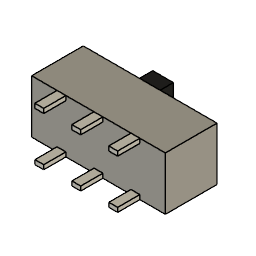
olliebella v1 extended (Autodesk Fusion 360 archive; units mm, degrees)
design "MSK-1153 slide switch SLV"
Autodesk Fusion 360 part; units mm, degrees
note: some values were not read from the file. Chosen so that the rebuilt part matches the saved one: which bodies a step acts on; which face or edge a step refers to.
sketch "Sketch1" plane through (0, 0, 0) normal (0, 0, 1) x (1, 0, 0)
  line L0 (-4.525, 3.5) -> (4.525, 3.5)
  line L1 (4.525, 3.5) -> (4.525, 0)
  line L2 (4.525, 0) -> (-4.525, 0)
  line L3 (-4.525, 0) -> (-4.525, 3.5)
  line L4 (-1.825, 5.5) -> (-0.425, 5.5)
  line L5 (-0.425, 5.5) -> (-0.425, 3.5)
  line L6 (-0.425, 3.5) -> (-1.825, 3.5)
  line L7 (-1.825, 3.5) -> (-1.825, 5.5)
  line L8 (-4.525, 0) -> (-4.525, -3.1) construction
  line L9 (-4.525, -3.1) -> (4.525, -3.1) construction
  line L10 (4.525, -3.1) -> (4.525, 0) construction
  line L11 (0, 0) -> (0, -3.1) construction
  line L12 (0.3, 0) -> (0.3, -3.1)
  line L13 (-0.3, -3.1) -> (-0.3, 0)
  line L14 (0.3, -1.55) -> (-0.3, -1.55) construction
  line L15 (-0.3, -3.1) -> (0.3, -3.1)
  line L16 (-2.8, 0) -> (-2.8, -3.1)
  line L17 (-2.2, -3.1) -> (-2.2, 0)
  line L18 (-2.5, 0) -> (-2.5, -3.1) construction
  line L19 (-2.8, -3.1) -> (-2.2, -3.1)
  line L20 (-2.8, -1.55) -> (-2.2, -1.55) construction
  line L21 (2.5, 0) -> (2.5, -3.1) construction
  line L22 (2.8, 0) -> (2.8, -3.1)
  line L23 (2.2, -3.1) -> (2.2, 0)
  line L24 (2.2, -1.55) -> (2.8, -1.55) construction
  line L25 (2.8, -3.1) -> (2.2, -3.1)
  line L26 (-2.025, 3.5) -> (-2.025, 2.9)
  line L27 (-2.025, 2.9) -> (2.025, 2.9)
  line L28 (2.025, 2.9) -> (2.025, 3.5)
  line L29 (-0.425, 5.5) -> (1.825, 5.5) construction
  line L30 (1.825, 5.5) -> (1.825, 3.5) construction
  dimension "d1" = 9.05
  dimension "d2" = 3.5
  dimension "d3" = 2
  dimension "d4" = 1.4
  dimension "d5" = 2.7
  dimension "d6" = 6.6
  dimension "d7" = 0.6
  dimension "d8" = 2.5
  dimension "d9" = 2.5
  dimension "d24" = 0.6
  dimension "d25" = 0.2
  dimension "d26" = 2.7
  dimension "d27" = 0.2
  constraint horizontal L0
  constraint vertical L1
  constraint horizontal L2
  constraint vertical L3
  constraint midpoint L11.start L2
  constraint horizontal L4
  constraint vertical L5
  constraint horizontal L6
  constraint vertical L7
  constraint coincident L0 L5.end
  constraint perpendicular L2 L8
  constraint perpendicular L1 L9
  constraint perpendicular L2 L10
  constraint coincident L11.start origin
  constraint midpoint L9 L11.end
  constraint coincident L2 L12.start
  constraint coincident L9 L12.end
  constraint coincident L9 L13.start
  constraint coincident L2 L13.end
  constraint vertical L13
  constraint vertical L12
  constraint midpoint L12 L14.start
  constraint midpoint L13 L14.end
  constraint midpoint L11 L14
  constraint coincident L2 L16.start
  constraint coincident L9 L16.end
  constraint coincident L9 L17.start
  constraint coincident L2 L17.end
  constraint vertical L17
  constraint vertical L16
  constraint coincident L2 L18.start
  constraint coincident L9 L18.end
  constraint perpendicular L9 L18
  constraint midpoint L16 L20.start
  constraint midpoint L17 L20.end
  constraint equal L14 L20
  constraint midpoint L18 L20
  constraint coincident L2 L21.start
  constraint coincident L9 L21.end
  constraint perpendicular L9 L21
  constraint coincident L2 L22.start
  constraint coincident L9 L22.end
  constraint coincident L9 L23.start
  constraint coincident L2 L23.end
  constraint vertical L23
  constraint vertical L22
  constraint midpoint L23 L24.start
  constraint midpoint L22 L24.end
  constraint midpoint L21 L24
  constraint equal L14 L24
  constraint coincident L0 L26.start
  constraint perpendicular L0 L26
  constraint perpendicular L26 L27
  constraint coincident L0 L28.end
  constraint perpendicular L0 L28
  constraint perpendicular L5 L29
  constraint coincident L0 L30.end
  constraint perpendicular L0 L30
  measures "d1" distance of L0.start L0.end
  measures "d2" distance of L0.start L2.end
  measures "d3" distance of L4 L6
  measures "d4" distance of L5 L7
  measures "d5" distance of L0.start L7
  measures "d6" distance of L0 L9
  measures "d7" distance of L14.start L14.end
  measures "d8" distance of L11 L18
  measures "d9" distance of L11 L21
  measures "d24" distance of L0 L27
  measures "d25" distance of L7 L26
  measures "d26" distance of L0.end L30
  measures "d27" distance of L28 L30
extrude "Extrude2" add sketch "Sketch1" along normal blind 1.8 and the other way blind 1.8 contours L0 L1 L2 L3 L26 L27 L28 | L0 L6 L26 L27 L28 makes body 1
extrude "Extrude1" add sketch "Sketch1" against normal blind 0.3 from surface at 1.8 separate body contours L2 L16 L17 L19 | L2 L12 L13 L15 | L2 L22 L23 L25 makes body 2 at (-2.6, -1.0333, 1.8) makes body 3 at (-0.1, -1.0333, 1.8) makes body 4 at (2.4, -1.0333, 1.8)
extrude "Extrude3" add sketch "Sketch1" along normal blind 0.3 from surface at -1.8 separate body contours L2 L16 L17 L19 | L2 L12 L13 L15 | L2 L22 L23 L25 makes body 5 at (-2.6, -1.0333, -1.8) makes body 6 at (-0.1, -1.0333, -1.8) makes body 7 at (2.4, -1.0333, -1.8)
extrude "Extrude4" add sketch "Sketch1" along normal blind 0.7 and the other way blind 0.7 separate body contours L0 L4 L5 L6 L7 makes body 8
extrude "Extrude5" add sketch "Sketch1" along normal up to surface (0.9 mm away) and the other way up to surface (0.9 mm away) separate body contours L0 L6 L26 L27 L28 makes body 9
combine "Combine1" operation cut target body 1 tool bodies 9 keep tools
move_body "Move1" bodies 9 to x (1, 0, 0) y (0, 1, 0) z (0, 0, 1) at (0, -0.2, 0)
extrude "Extrude6" add 1 faces at (-1.3583, 3.5, -0.2333) along direction (0, -1, 0) blind 0.5 on bodies 8 bodies 8 9
extrude "Extrude7" cut 1 faces at (-1.5083, 0, 0.6) along direction (0, -1, 0) up to surface (1.6 mm away) from surface at 1.5 on bodies 1 bodies 2 3 4 5 6 7

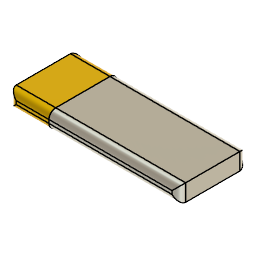
design "Lipo 100mAh 301230"
Autodesk Fusion 360 part; units mm, degrees
sketch "Sketch1" plane through (0, 0, 0) normal (0, 0, 1) x (1, 0, 0) in component "Lipo_Body"
  line L0 (15, -6) -> (-15, -6)
  line L1 (-15, -6) -> (-15, 6)
  line L2 (-15, 6) -> (15, 6)
  line L3 (15, 6) -> (15, -6)
  line L4 (15, -6) -> (-15, 6) construction
  line L5 (-15, -6) -> (15, 6) construction
  line L6 (-8, 6) -> (-8, -6)
  dimension "d1" = 30
  dimension "d3" = 7
  dimension "d74" = 12
  constraint horizontal L0
  constraint perpendicular L0 L1
  constraint parallel L0 L2
  constraint parallel L1 L3
  constraint coincident L4 origin
  constraint coincident L5 origin
  constraint coincident L2 L6.start
  constraint coincident L0 L6.end
  constraint perpendicular L0 L6
  measures "d1" distance of L1.end L2.end
  measures "d3" distance of L1 L6
  measures "d74" distance of L0 L2
extrude "Extrude1" add sketch "Sketch1" along normal blind 3 contours L0 L2 L3 L6 makes body 1 in component "Lipo_Body"
extrude "Extrude2" add sketch "Sketch1" along normal up to surface (3 mm away) separate body contours L0 L1 L2 L6 makes body 2 in component "Lipo_Body"
fillet "Fillet1" radius 1.2 12 edges at (15, -6, 1.5) (15, 6, 1.5) (3.5, -6, 3) (3.5, -6, 0) (3.5, 6, 3) (3.5, 6, 0) (-15, -6, 1.5) (-15, 6, 1.5) (-11.5, -6, 3) (-11.5, -6, 0) (-11.5, 6, 3) (-11.5, 6, 0) on bodies 1 2 in component "Lipo_Body"
shell "Shell2" [suppressed] in component "Lipo_Body"
component "Lipo_Body" placed x (1, 0, 0) y (0, 1, 0) z (0, 0, 1) at (0, 0, 0)
equation "d5_1 = 0.1 mm + 0.05 mm"
equation "d9_1 = 0.1 mm - 0.05 mm"
equation "d13_1 = ( 2.8 / 2 ) * 1 mm"
equation "d19_1 = ( 1.9 / 2 ) * 1 mm"
equation "d20_1 = ( -1.9 / 2 ) * 1 mm"
equation "d13_2 = ( 2.8 / 2 ) * 1 mm"
equation "d19_2 = ( 1.9 / 2 ) * 1 mm"
equation "d20_2 = ( -1.9 / 2 ) * 1 mm"
equation "d80 = 1.6 mm - 0.3 mm"
named bodies: "sticker"

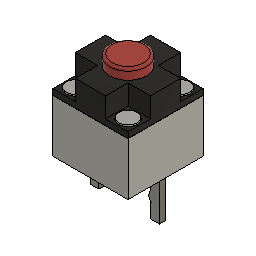
design "kailh cmi627301D07"
Autodesk Fusion 360 part; units mm, degrees
ref_plane "WorkPlane1" through (0, 0, 10) normal (0, 0, 1) x (1, 0, 0)
ref_plane "WorkPlane2" through (0, 0, 3.5) normal (0, 0, 1) x (1, 0, 0)
ref_plane "WorkPlane3" through (0, 0, 0.2) normal (0, 0, 1) x (1, 0, 0)
sketch "top" plane through (0, 0, 10) normal (0, 0, 1) x (1, 0, 0)
  line L0 (0, 0) -> (0, 5) construction
  line L1 (3.1, 8.1) -> (-3.1, 8.1)
  line L2 (-3.1, 8.1) -> (-3.1, 1.9)
  line L3 (-3.1, 1.9) -> (3.1, 1.9)
  line L4 (3.1, 1.9) -> (3.1, 8.1)
  line L5 (3.1, 8.1) -> (-3.1, 1.9) construction
  line L6 (-3.1, 8.1) -> (3.1, 1.9) construction
  circle A0 centre (0, 5) radius 1.5
  line L7 (-3.1, 6.25) -> (3.1, 6.25) construction
  line L8 (3.1, 3.75) -> (-3.1, 3.75) construction
  line L9 (-1.25, 8.1) -> (-1.25, 1.9) construction
  line L10 (1.25, 1.9) -> (1.25, 8.1) construction
  line L11 (1.25, 6.25) -> (-1.25, 3.75) construction
  line L12 (-1.25, 8.1) -> (-1.25, 6.25)
  line L13 (-3.1, 6.25) -> (-1.25, 6.25)
  line L14 (1.25, 6.25) -> (1.25, 8.1)
  line L15 (1.25, 6.25) -> (3.1, 6.25)
  line L16 (1.25, 3.75) -> (3.1, 3.75)
  line L17 (1.25, 3.75) -> (1.25, 1.9)
  line L18 (-1.25, 3.75) -> (-1.25, 1.9)
  line L19 (-1.25, 3.75) -> (-3.1, 3.75)
  line L20 (1.25, 3.75) -> (3.1, 1.9) construction
  line L21 (1.25, 6.25) -> (3.1, 8.1) construction
  line L22 (-1.25, 6.25) -> (-3.1, 8.1) construction
  line L23 (-1.25, 3.75) -> (-3.1, 1.9) construction
  circle A1 centre (2.175, 2.825) radius 0.75
  circle A2 centre (-2.175, 2.825) radius 0.75
  circle A3 centre (-2.175, 7.175) radius 0.75
  circle A4 centre (2.175, 7.175) radius 0.75
  point P0 (0, 5)
  dimension "d3" = 5
  dimension "d4" = 6.2
  dimension "d5" = 6.2
  dimension "d6" = 3
  dimension "d7" = 2.5
  dimension "d8" = 2.5
  dimension "d19" = 1.5
  constraint coincident L0.start origin
  constraint vertical L0
  constraint horizontal L1
  constraint perpendicular L1 L2
  constraint parallel L1 L3
  constraint parallel L2 L4
  constraint coincident L5 P0
  constraint coincident L6 P0
  constraint coincident P0 L0.end
  constraint coincident L2 L7.start
  constraint coincident L4 L7.end
  constraint perpendicular L4 L7
  constraint coincident L4 L8.start
  constraint coincident L2 L8.end
  constraint perpendicular L2 L8
  constraint coincident L1 L9.start
  constraint coincident L3 L9.end
  constraint perpendicular L3 L9
  constraint coincident L3 L10.start
  constraint coincident L1 L10.end
  constraint perpendicular L1 L10
  constraint coincident L10 L11.start
  constraint coincident L7 L11.start
  constraint coincident L8 L11.end
  constraint coincident L9 L11.end
  constraint midpoint P0 L11
  constraint coincident L7 L12.end
  constraint coincident L9 L12.end
  constraint coincident L8 L16.start
  constraint coincident L6 L16.start
  constraint midpoint L20 A1.centre
  constraint midpoint L23 A2.centre
  constraint midpoint L22 A3.centre
  constraint midpoint L21 A4.centre
  constraint equal A1 A2
  constraint equal A2 A3
  constraint equal A3 A4
  measures "d3" distance of L0.start P0
  measures "d4" distance of L2.end L3.end
  measures "d5" distance of L1.end L2.end
  measures "d6" diameter of A0
  measures "d7" distance of L9 L10
  measures "d8" distance of L7 L8
  measures "d19" diameter of A1
extrude "Extrude1" add sketch "top" against normal up to surface (6.5 mm away) contours L1 L4 L14 L15 | L1 L2 L3 L4 L12 L13 L14 L15 L16 L17 L18 L19 | L1 L2 L12 L13 | L3 L4 L16 L17 | L2 L3 L18 L19 | A0 | A1 | A2 | A3 | A4 makes body 1
extrude "Extrude2" cut sketch "top" against normal blind 1.65 contours L1 L4 L14 L15 | L1 L2 L12 L13 | L3 L4 L16 L17 | L2 L3 L18 L19 | A1 | A2 | A3 | A4 bodies 1
extrude "Extrude3" add sketch "top" along normal blind 0.85 separate body contours A0 makes body 2
ref_plane "WorkPlane4" through (2.175, 7.175, 7.85) normal (0, 0, 1) x (1, 0, 0)
split "Split1" by plane through (2.175, 7.175, 7.85) normal (0, 0, 1) bodies 1 makes body 3 at (-0.4167, 5.4167, 10)
extrude "Extrude5" cut sketch "top" against normal up to surface (2.15 mm away) contours A1 | A2 | A3 | A4 bodies 3
move_face "OffsetFaces1" offset -0.02 5 faces at (2.9213, 7.1003, 8.1833) (2.9213, 2.7503, 8.1833) (-1.4287, 7.1003, 8.1833) (-1.4287, 2.7503, 8.1833) (-0.5417, 5.555, 7.85) on bodies 3
extrude "Extrude6" add sketch "top" along normal up to surface (0.6 mm away) from surface at -2.15 contours A1 | A2 | A3 | A4 bodies 1
fillet "Fillet1" radius 0.2 1 edges at (-1.3985, 4.4576, 10.85) on bodies 2
sketch "bottom" plane through (0, 0, 3.5) normal (0, 0, -1) x (1, 0, 0)
  line L0 (-3.1, -8.1) -> (3.1, -8.1)
  line L1 (3.1, -8.1) -> (3.1, -1.9)
  line L2 (3.1, -1.9) -> (-3.1, -1.9)
  line L3 (-3.1, -1.9) -> (-3.1, -8.1)
  line L4 (-3.1, -5) -> (3.1, -5) construction
  line L5 (-2.5, -5) -> (2.5, -5) construction
  circle A0 centre (2.5, -5) radius 0.55 construction
  circle A1 centre (-2.5, -5) radius 0.55 construction
  dimension "d17" = 5
  dimension "d18" = 1.1
  constraint midpoint L3 L4.start
  constraint midpoint L1 L4.end
  constraint coincident L5.end A0.centre
  constraint coincident L5.start A1.centre
  constraint equal A0 A1
  constraint parallel L4 L5
  constraint midpoint L4 L5
  measures "d17" distance of L5.start L5.end
  measures "d18" diameter of A0
ref_plane "WorkPlane5" through (0, 5, 3.5) normal (0, -1, 0) x (1, 0, 0)
sketch "pin" plane through (0, 5, 0) normal (0, -1, 0) x (-1, 0, 0)
  line L0 (2.5, -3.5) -> (-2.5, -3.5)
  line L1 (-1.95, -3.5) -> (-3.05, -3.5)
  line L2 (-2.15, -3.5) -> (-2.85, -3.5)
  line L3 (-2.85, -3.5) -> (-2.85, -0.2)
  line L4 (-2.85, -0.2) -> (-2.15, -0.2)
  line L5 (-2.15, -0.2) -> (-2.15, -3.5) construction
  line L6 (3.1, -3.5) -> (-3.1, -3.5)
  line L7 (-2.5, -3.5) -> (-2.5, -0.2) construction
  line L8 (-2.15, -0.2) -> (-2.15, -1.4)
  line L9 (-2.15, -1.4) -> (-1.95, -1.8)
  line L10 (-1.95, -1.8) -> (-2.15, -2.5)
  line L11 (-2.15, -3.5) -> (-2.15, -2.5)
  line L12 (-1.95, -1.8) -> (-2.85, -1.8) construction
  line L13 (3.1, -3.5) -> (-3.1, -3.5)
  line L14 (0, -3.5) -> (0, 0) construction
  point P0 (-2.5, -3.5)
  dimension "d37" = 0.7
  dimension "d38" = 3.3
  dimension "d39" = 0.9
  dimension "d40" = 1.7
  dimension "d42" = 0.4
  dimension "d43" = 0.7
  constraint coincident L0 L2.start
  constraint coincident L1 L2.end
  constraint perpendicular L2 L3
  constraint perpendicular L3 L4
  constraint parallel L3 L5
  constraint midpoint L2 P0
  constraint coincident P0 L0.end
  constraint midpoint L4 L7.end
  constraint coincident L5 L8.end
  constraint coincident L5 L10.end
  constraint coincident L3 L12.end
  constraint perpendicular L3 L12
  constraint midpoint L0 L14.start
  constraint coincident L14.end origin
  measures "d37" distance of L3.end L4.end
  measures "d38" distance of L4 L6
  measures "d39" distance of L9.end L12.end
  measures "d40" distance of L12 L13
  measures "d42" distance of L8.end L12
  measures "d43" distance of L10.end L12
extrude "Extrude8" add sketch "pin" along normal mid plane 0.5 separate body makes body 4
mirror "Mirror2" about plane through (0, 0, 0) normal (1, 0, 0) of bodies 4 makes body 5
equation "d11 = -( 6.5 mm - 4.85 mm )"
named bodies: "case", "cover", "cap", "pin", "pin (1)"

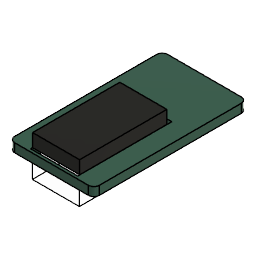
design "paw3950-surface"
Autodesk Fusion 360 part; units mm, degrees
ref_plane "WorkPlane1" through (0, 0, 4.1) normal (0, 0, 1) x (1, 0, 0)
sketch "PAW3395 breakout" plane through (0, 0, 4.1) normal (0, 0, 1) x (1, 0, 0)
  line L0 (7.8, -9.4) -> (-7.8, -9.4) construction
  line L1 (-7.8, -9.4) -> (-7.8, 18.7) construction
  line L2 (7.8, 18.7) -> (7.8, -9.4) construction
  line L3 (-7.8, 18.7) -> (7.8, 18.7) construction
  line L4 (0, 18.7) -> (0, -9.4) construction
  line L5 (0, 0) -> (0, -9.4) construction
  line L6 (-4.3, 8.35) -> (4.3, 8.35)
  line L7 (4.3, 8.35) -> (4.3, -8.83)
  line L8 (4.3, -8.83) -> (-4.3, -8.83)
  line L9 (-4.3, -8.83) -> (-4.3, 8.35)
  line L10 (0, 8.35) -> (0, -8.83) construction
  line L11 (-4.3, 7.45) -> (4.3, 7.45)
  line L12 (-4.3, -8.55) -> (4.3, -8.55)
  line L13 (4.3, 7.65) -> (-4.3, 7.65)
  line L14 (-4.3, -8.5) -> (4.3, -8.5)
  circle A0 centre (6.8, 17.7) radius 1 construction
  circle A1 centre (-6.8, 17.7) radius 1 construction
  circle A2 centre (6.8, -8.4) radius 1 construction
  circle A3 centre (-6.8, -8.4) radius 1 construction
  line L15 (-6.8, 18.7) -> (6.8, 18.7)
  line L16 (7.8, 17.7) -> (7.8, -8.4)
  line L17 (6.8, -9.4) -> (-6.8, -9.4)
  line L18 (-7.8, -8.4) -> (-7.8, 17.7)
  arc A4 (7.8, 17.7) -> (6.8, 18.7) centre (6.8, 17.7) ccw
  arc A5 (-6.8, 18.7) -> (-7.8, 17.7) centre (-6.8, 17.7) ccw
  arc A6 (-7.8, -8.4) -> (-6.8, -9.4) centre (-6.8, -8.4) ccw
  arc A7 (6.8, -9.4) -> (7.8, -8.4) centre (6.8, -8.4) ccw
  dimension "d3" = 15.6
  dimension "d579" = 28.1
  dimension "d584" = 0.57
  dimension "d585" = 17.18
  dimension "d586" = 8.6
  dimension "d725" = 3.5
  dimension "d726" = 3.5
  dimension "d728" = 2
  dimension "d815" = 0.85
  dimension "d816" = 0.9
  dimension "d845" = 9.4
  dimension "d850" = 15.95
  constraint horizontal L3
  constraint vertical L2
  constraint horizontal L0
  constraint midpoint L0 L4.end
  constraint vertical L5
  constraint horizontal L6
  constraint vertical L7
  constraint horizontal L8
  constraint vertical L9
  constraint midpoint L6 L10.start
  constraint midpoint L8 L10.end
  constraint collinear L4 L10
  constraint coincident L9 L11.start
  constraint coincident L7 L11.end
  constraint perpendicular L7 L11
  constraint coincident L9 L12.start
  constraint coincident L7 L12.end
  constraint perpendicular L7 L12
  constraint coincident L7 L13.start
  constraint coincident L9 L13.end
  constraint perpendicular L9 L13
  constraint coincident L9 L14.start
  constraint coincident L7 L14.end
  constraint perpendicular L7 L14
  constraint coincident L0 L4.end
  constraint coincident L5.start origin
  constraint midpoint L3 L4.start
  constraint tangent L3 A0
  constraint tangent L2 A0
  constraint tangent L3 A1
  constraint tangent L1 A1
  constraint equal A0 A1
  constraint tangent L2 A2
  constraint tangent L0 A2
  constraint tangent L0 A3
  constraint tangent L1 A3
  constraint equal A2 A3
  constraint equal A0 A2
  constraint coincident A1 L15.start
  constraint coincident L3 L15.start
  constraint coincident A0 L15.end
  constraint coincident L3 L15.end
  constraint coincident A0 L16.start
  constraint coincident L2 L16.start
  constraint coincident L2 L16.end
  constraint coincident A2 L16.end
  constraint coincident L0 L17.start
  constraint coincident A2 L17.start
  constraint coincident L0 L17.end
  constraint coincident A3 L17.end
  constraint coincident A3 L18.start
  constraint coincident L1 L18.start
  constraint coincident A1 L18.end
  constraint coincident L1 L18.end
  constraint tangent L15 A4
  constraint tangent L18 A5
  constraint tangent L18 A6
  constraint tangent L17 A7
  constraint tangent L16 A7
  constraint coincident L5.start L4
  measures "d3" distance of L1.end L2.start
  measures "d579" distance of L0 L3
  measures "d584" distance of L0 L8
  measures "d585" distance of L6 L8
  measures "d586" distance of L7 L9
  measures "d725" distance of L2 L7
  measures "d726" distance of L1 L9
  measures "d728" diameter of A0
  measures "d815" distance of L12 L17
  measures "d816" distance of L14 L17
  measures "d845" distance of L5.start L17
  measures "d850" distance of L11 L14
  measures "d851" distance of L12 L13
extrude "Extrude1" add sketch "PAW3395 breakout" along normal blind 1.6 makes body 1
move_face "OffsetFaces21" offset -0.05 4 faces at (7.8, 9, 4.6333) (-7.8, 0.3, 4.6333) (2.2667, -9.4, 4.6333) (-2.2667, 18.7, 4.6333) on bodies 1
ref_plane "WorkPlane2" through (0, 4.65, 0.7) normal (0, 0, -1) x (-1, 0, 0)
extrude "Extrude81" add sketch "PAW3395 breakout" against normal up to surface (3.38 mm away) from surface at -0.01 separate body contours L7 L9 L11 L13 | L7 L9 L11 L14 | L7 L9 L12 L14 makes body 2
ref_plane "WorkPlane14" through (0, 4.65, 8.1) normal (0, 0, 1) x (1, 0, 0)
extrude "Extrude82" add sketch "PAW3395 breakout" along normal up to surface (2.39 mm away) from surface at 1.61 separate body contours L7 L9 L11 L14 makes body 3
sketch "mount core" plane through (0, 0, 0.7) normal (0, 0, -1) x (-1, 0, 0)
  line L0 (7.8, -9.4) -> (7.8, 18.7)
  line L1 (-7.8, 18.7) -> (7.8, 18.7)
  line L2 (7.8, -9.4) -> (-7.8, -9.4)
  line L3 (-7.8, 18.7) -> (-7.8, -9.4)
  line L4 (4.3, -7.95) -> (-4.3, -7.95)
  arc A0 (6.8, -9.4) -> (7.8, -8.4) centre (6.8, -8.4) ccw
  line L5 (3.7, -7.95) -> (3.7, 7.05)
  line L6 (-3.7, -7.95) -> (-3.7, 7.05)
  line L7 (4.3, -8.55) -> (4.3, 7.65)
  line L8 (-4.3, 7.65) -> (-4.3, -8.55)
  line L9 (4.3, 7.05) -> (-4.3, 7.05)
  line L10 (4.3, 7.65) -> (-4.3, 7.65)
  line L11 (5.1, -9.35) -> (-5.1, -9.35)
  line L12 (-5.1, -9.35) -> (-5.1, 8.45)
  line L13 (-5.1, 8.45) -> (5.1, 8.45)
  line L14 (5.1, 8.45) -> (5.1, -9.35)
  line L15 (4.3, -8.55) -> (-4.3, -8.55)
  dimension "d822" = 0.6
  dimension "d823" = 0.6
  dimension "d824" = 0.6
  dimension "d825" = 0.6
  dimension "d826" = 0.8
  dimension "d827" = 0.8
  dimension "d828" = 0.8
  dimension "d829" = 0.8
  dimension "d851" = 16.2
  constraint coincident L4 L5.start
  constraint coincident L4 L6.start
  constraint coincident L4.start L7
  constraint coincident L4.end L8
  constraint coincident L7 L9.start
  constraint coincident L8 L9.end
  constraint perpendicular L8 L9
  constraint coincident L5.end L9
  constraint coincident L6.end L9
  constraint parallel L2 L11
  constraint perpendicular L11 L12
  constraint perpendicular L12 L13
  constraint perpendicular L11 L14
  measures "d822" distance of L4 L15
  measures "d823" distance of L6 L8
  measures "d824" distance of L5 L7
  measures "d825" distance of L9 L10
  measures "d826" distance of L7 L14
  measures "d827" distance of L10 L13
  measures "d828" distance of L8 L12
  measures "d829" distance of L11 L15
ref_plane "WorkPlane19" through (0, 4.65, 0) normal (0, 0, -1) x (-1, 0, 0)
equation "d1 = dis_len_to_surface + 3.4 mm"
equation "d817 = dis_len_to_surface"
equation "dis_len_to_surface = 0.7 mm"
equation "d685 = ball_dia / 2"
equation "d693 = ball_dia / 2"
equation "d695 = ball_dia / 2"
equation "d698 = ball_dia / 2"
equation "ball_dia_1 = 40 mm"
named bodies: "PMW3610 breakout", "PMW3610 lens", "PMW3610 sensor"
